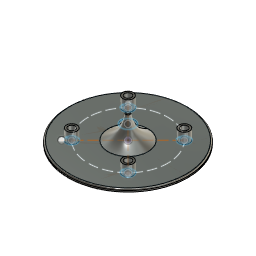
Bottom cover (Autodesk Fusion 360 design; units mm, degrees)
Autodesk Fusion 360 part; units mm, degrees
note: some values were not read from the file. Set by a fixed rule: which sketch regions a step uses.
sketch "Sketch1" plane through (0, 0, 0) normal (1, 0, 0) x (0, 1, 0)
  line L0 (0, 80) -> (0, -40) construction
  line L1 (0, 0) -> (45, 0)
  line L2 (45, 0) -> (45, 1)
  line L3 (0, 0) -> (0, 20) construction
  line L4 (0, 20) -> (1.5, 20)
  line L5 (44, 2) -> (15, 2)
  spline S0 degree 2 poles (1.5, 20) (4.0396, 7.8722) (15, 2) knots 0 0 0 2.340033 2.340033 2.340033 weights 1 1.582771 1
  arc A0 (45, 1) -> (44, 2) centre (44, 1) ccw
  line L6 (0, 20) -> (0, 0) construction
  line L7 (0, 20) -> (0, 0)
  point P0 (45, 2)
  dimension "d1" = 120
  dimension "d2" = 45
  dimension "d3" = 2
  dimension "d4" = 20
  dimension "d5" = 1.5
  dimension "d6" = 30
  dimension "d7" = 1
  constraint vertical L0
  constraint coincident L1.start L3.start
  constraint perpendicular L0 L1
  constraint perpendicular L1 L2
  constraint perpendicular L1 L3
  constraint horizontal L4
  constraint perpendicular L2 L5
  constraint coincident P0 L2
  constraint coincident P0 L5
  constraint tangent L2 A0
  constraint tangent L5 A0
  measures "d1" distance of L0.start L0.end
  measures "d2" distance of L1.start L1.end
  measures "d3" distance of L1.end P0
  measures "d4" distance of L1.start L3.end
  measures "d5" distance of L3.end L4.end
  measures "d6" distance of P0 L5.end
  measures "d7" radius of A0
revolve "Revolve1" add sketch "Sketch1" angle 360 about axis through (0, 0, 20) along (0, 0, -1)
fillet "Fillet1" radius 0.5 1 edges at (-1.3985, 0.5424, 20)
sketch "Sketch2" plane through (0, 0, 2) normal (0, 0, 1) x (-1, 0, 0)
  circle A0 centre (0, 0) radius 15
  circle A1 centre (0, 0) radius 44
  circle A2 centre (0, 0) radius 30 construction
  line L0 (0, 0) -> (25, 25) construction
  line L1 (0, 0) -> (-21.2132, -21.2132) construction
  line L2 (0, 0) -> (-22.657, 22.657) construction
  line L3 (0, 0) -> (23.9132, -23.9132) construction
  circle A3 centre (21.2132, -21.2132) radius 4
  circle A4 centre (-21.2132, -21.2132) radius 4
  circle A5 centre (21.2132, 21.2132) radius 4
  circle A6 centre (-21.2132, 21.2132) radius 4
  circle A7 centre (21.2132, -21.2132) radius 2.6
  circle A8 centre (-21.2132, -21.2132) radius 2.6
  circle A9 centre (-21.2132, 21.2132) radius 2.6
  circle A10 centre (21.2132, 21.2132) radius 2.6
  circle A11 centre (10.6066, -10.6066) radius 5
  dimension "d11" = 60
  dimension "d12" = 35.3553
  dimension "d13" = 30
  dimension "d14" = 32.0419
  dimension "d15" = 33.8184
  dimension "d16" = 8
  dimension "d17" = 8
  dimension "d18" = 8
  dimension "d19" = 8
  dimension "d20" = 5.2
  dimension "d21" = 5.2
  dimension "d22" = 5.2
  dimension "d23" = 5.2
  dimension "d31" = 10
  dimension "d34" = 15
  constraint coincident A0.centre A1.centre
  constraint coincident A2 L1.end
  constraint parallel L0 L1
  constraint perpendicular L1 L2
  constraint perpendicular L1 L3
  constraint coincident A2 A3.centre
  constraint coincident L3 A3.centre
  constraint coincident L1.end A4.centre
  constraint coincident A2 A5.centre
  constraint coincident L0 A5.centre
  constraint coincident A2 A6.centre
  constraint coincident L2 A6.centre
  constraint concentric A3 A7
  constraint concentric A4 A8
  constraint concentric A6 A9
  constraint concentric A5 A10
  constraint coincident L3 A11.centre
  constraint coincident A0 A11.centre
  measures "d11" diameter of A2
  measures "d12" distance of A0.centre L0.end
  measures "d13" distance of A0.centre L1.end
  measures "d14" distance of A0.centre L2.end
  measures "d15" distance of A0.centre L3.end
  measures "d16" diameter of A3
  measures "d17" diameter of A4
  measures "d18" diameter of A5
  measures "d19" diameter of A6
  measures "d20" diameter of A7
  measures "d21" diameter of A8
  measures "d22" diameter of A9
  measures "d23" diameter of A10
  measures "d31" diameter of A11
  measures "d34" distance of A3.centre A11.centre
extrude "Extrude3" add sketch "Sketch2" along normal blind 8 contours A3 | A4 | A5 | A6
extrude "Extrude2" cut sketch "Sketch2" against normal blind 5 contours A7 | A8 | A9 | A10
extrude "Extrude4" cut sketch "Sketch2" along normal mid plane 18 contours A0 A11 | A0 A11 picked at (9.3285, -9.5024) picked at (11.819, -11.7173)
